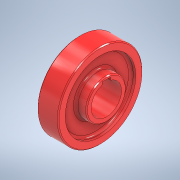
# Autodesk Inventor part: звездочка
Saved by Autodesk Inventor 2021 (Build 250183000, 183)
## iProperties
Created: 2023-04-24
Part Number: звездочка
Material: Сталь, углеродистая
Document SubType Name: Modeling
Designer: gdevc
Density: 7.85 g/cm^3
Appearance: Светло-красный
Author: gdevc
Autodesk Inventor part; units mm, degrees
ref_plane "YZ Plane" through (0, 0, 0) normal (1, 0, 0) x (0, 1, 0)
ref_plane "XY Plane" through (0, 0, 0) normal (0, 0, 1) x (1, 0, 0)
sketch "Эскиз1" plane through (0, 0, 0) normal (0, 0, 1) x (1, 0, 0)
  line L0 (0, 32.5) -> (70, 32.5)
  line L1 (0, 0) -> (109.6934, 0)
  line L2 (0, 32.5) -> (0, 40.5)
  line L3 (35, 68.0113) -> (35, 17.7812) construction
  line L4 (0, 80) -> (70, 80) construction
  line L5 (14.5, 90.75) -> (55.5, 90.75)
  line L6 (12.5, 75.5) -> (18.0123, 75.5)
  line L7 (2, 42.5) -> (18.0123, 42.5)
  line L8 (23.0123, 47.5) -> (23.0123, 70.5)
  arc A0 (18.0123, 42.5) -> (23.0123, 47.5) centre (18.0123, 47.5) ccw
  arc A1 (23.0123, 70.5) -> (18.0123, 75.5) centre (18.0123, 70.5) ccw
  line L9 (12.5, 75.5) -> (12.5, 88.75)
  line L10 (70, 32.5) -> (0, 32.5)
  line L11 (70, 32.5) -> (70, 40.5)
  line L12 (57.5, 90.75) -> (12.5, 90.75)
  line L13 (57.5, 75.5) -> (51.9877, 75.5)
  line L14 (68, 42.5) -> (51.9877, 42.5)
  line L15 (46.9877, 47.5) -> (46.9877, 70.5)
  arc A2 (46.9877, 47.5) -> (51.9877, 42.5) centre (51.9877, 47.5) ccw
  arc A3 (51.9877, 75.5) -> (46.9877, 70.5) centre (51.9877, 70.5) ccw
  line L16 (57.5, 75.5) -> (57.5, 88.75)
  line L17 (12.5, 88.75) -> (14.5, 90.75)
  line L18 (55.5, 90.75) -> (57.5, 88.75)
  line L19 (0, 40.5) -> (2, 42.5)
  line L20 (68, 42.5) -> (70, 40.5)
  point P0 (0, 42.5)
  point P1 (12.5, 90.75)
  point P2 (57.5, 90.75)
  point P3 (70, 42.5)
  dimension "d0" = 65
  dimension "d1" = 70
  dimension "d2" = 160
  dimension "d3" = 181.5
  dimension "d4" = 151
  dimension "d5" = 85
  dimension "d6" = 5
  dimension "d7" = 5
  dimension "d8" = 45
  dimension "d9" = 45
  dimension "d10" = 70
  dimension "d11" = 2
  dimension "d12" = 2
  dimension "d13" = 2
  dimension "d14" = 2
  dimension "d15" = 2
  dimension "d16" = 2
  dimension "d17" = 2
  dimension "d18" = 2
  constraints: 42 end point, 12 symmetric about line, 11 point on line, 8 point on circle, 6 horizontal, 4 centre point, 4 tangent, 3 vertical, 1 perpendicular, 2 other
  measures "d0" diameter of L0 L1
  measures "d1" distance of L0.start L0.end
  measures "d2" diameter of L4 L1
  measures "d3" diameter of L5 L1
  measures "d4" diameter of L6 L1
  measures "d5" diameter of L7 L1
  measures "d6" radius of A0
  measures "d7" radius of A1
  measures "d8" diameter of L6.start L3
  measures "d9" distance of point (12.5, 90.75) point (57.5, 90.75)
  measures "d10" distance between parallel lines of L2 L11
  measures "d11" distance of L9.end point (12.5, 90.75)
  measures "d12" distance of L5.start point (12.5, 90.75)
  measures "d13" distance of L5.end point (57.5, 90.75)
  measures "d14" distance of L16.end point (57.5, 90.75)
  measures "d15" distance of L2.end point (0, 42.5)
  measures "d16" distance of L7.start point (0, 42.5)
  measures "d17" distance of L14.start point (70, 42.5)
  measures "d18" distance of L11.end point (70, 42.5)
revolve "Вращение1" add sketch "Эскиз1" angle 360 about axis through (0, 0, 0) along (1, 0, 0)
ref_plane "РабПлоскость1" through (0, 32.5, 0) normal (0, 1, 0) x (-1, 0, 0)
sketch "Эскиз2" plane through (0, 32.5, 0) normal (0, 1, 0) x (-1, 0, 0)
  line L0 (-70, -8.9471) -> (0, -8.9471)
  line L1 (0, -8.9471) -> (0, 9.0529)
  line L2 (0, 9.0529) -> (-70, 9.0529)
  line L3 (-70, 9.0529) -> (-70, -8.9471)
  line L4 (-70, 32.5) -> (-70, -32.5) projected
  point P0 (0, 0)
  dimension "d21" = 18
  dimension "d22" = 0
  dimension "d23" = 70
  constraints: 8 end point, 2 parallel, 1 horizontal, 1 perpendicular
  measures "d21" distance between parallel lines of L2 L0
  measures "d22" distance between parallel lines of L4 L3
  measures "d23" distance between parallel lines of L1 L3
extrude "Выдавливание1" cut sketch "Эскиз2" along normal blind 4.4 and the other way blind 19.45
equation "\"d12\" = d11"
equation "\"d13\" = d11"
equation "\"d14\" = d13"
equation "\"d15\" = d11"
equation "\"d16\" = d15"
equation "\"d17\" = d11"
equation "\"d18\" = d17"
